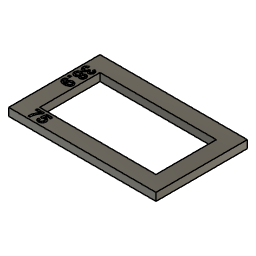
Test_Monitor (Autodesk Fusion 360 design; units mm, degrees)
Autodesk Fusion 360 part; units mm, degrees
sketch "Esboço1" plane through (0, 0, 0) normal (0, 0, 1) x (1, 0, 0)
  line L0 (37.5, -19.45) -> (-37.5, -19.45)
  line L1 (-37.5, -19.45) -> (-37.5, 19.45)
  line L2 (-37.5, 19.45) -> (37.5, 19.45)
  line L3 (37.5, 19.45) -> (37.5, -19.45)
  line L4 (37.5, -19.45) -> (-37.5, 19.45) construction
  line L5 (-37.5, -19.45) -> (37.5, 19.45) construction
  line L6 (-47.5, 29.45) -> (47.5, 29.45)
  line L7 (47.5, 29.45) -> (47.5, -29.45)
  line L8 (47.5, -29.45) -> (-47.5, -29.45)
  line L9 (-47.5, -29.45) -> (-47.5, 29.45)
  line L10 (-37.4956, -29.4613) -> (-11.7884, -29.45) construction
  line L11 (-11.7884, -29.45) -> (-11.7928, -19.4387) construction
  line L12 (-11.7928, -19.4387) -> (-37.5, -19.45) construction
  line L13 (-37.5, -19.45) -> (-37.4956, -29.4613) construction
  line L14 (-47.5394, 19.3771) -> (-47.4606, 8.5302) construction
  line L15 (-47.4606, 8.5302) -> (-37.4213, 8.6031) construction
  line L16 (-37.4213, 8.6031) -> (-37.5, 19.45) construction
  line L17 (-37.5, 19.45) -> (-47.5394, 19.3771) construction
  dimension "d1" = 75
  dimension "d2" = 38.9
  dimension "d3" = -10
  dimension "d6" = 7
  dimension "d7" = 7
  text T0 "75" font "Arial" height 7 bold align left middle in box 25.7072 x 10.0113 at (-37.4956, -29.4613) x (1, 0.00044) y (-0.00044, 1) spacing 1
  text T1 "38.9" font "Arial" height 7 bold align left middle in box 10.8472 x 10.0396 at (-47.5394, 19.3771) x (0.007258, -0.999974) y (0.999974, 0.007258) spacing 1
  constraint horizontal L0
  constraint perpendicular L0 L1
  constraint parallel L0 L2
  constraint parallel L1 L3
  constraint coincident L4 origin
  constraint coincident L5 origin
  constraint coincident L8
  constraint coincident L0.end
  constraint coincident L1.end
  constraint coincident L9
  measures "d1" distance of L1.end L2.end
  measures "d2" distance of L0.end L1.end
extrude "Extrusão1" add sketch "Esboço1" along normal blind 5
extrude "Extrusão2" cut sketch "Esboço1" against normal blind 1 from surface at 5 text T1 T0
equation "d4 = 5 mm"
equation "d10 = d4"
